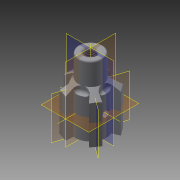
# Autodesk Inventor part: RadAxe
Saved by Autodesk Inventor 2015 (Build 190159000, 159)
## iProperties
Created: 2018-11-03
Part Number: RadAxe
Material: Generisch
Document SubType Name: Modeling
Designer: Boris
Density: 1 g/cm^3
Appearance: Vorgabe
Author: Boris
Autodesk Inventor part; units mm, degrees
sketch "Skizze1" plane through (0, 0, 0) normal (0, 0, 1) x (1, 0, 0)
  line L0 (0, -50.4) -> (0, 50.4)
  line L1 (50.4, 0) -> (-50.4, 0)
  line L2 (-7, 1.5) -> (-4.7724, 1)
  line L3 (-7, -1.5) -> (-4.7724, -1)
  line L4 (-7, -1.5) -> (-7, 1.5)
  line L5 (-0.7365, -7.1209) -> (-3.5897, -6.1939)
  line L6 (-0.7365, -7.1209) -> (-0.5237, -4.8478)
  line L7 (-3.5897, -6.1939) -> (-2.4258, -4.2298)
  line L8 (6.5448, -2.901) -> (4.7814, -5.328)
  line L9 (6.5448, -2.901) -> (4.4487, -1.9961)
  line L10 (4.7814, -5.328) -> (3.2731, -3.6141)
  line L11 (4.7814, 5.328) -> (6.5448, 2.901)
  line L12 (4.7814, 5.328) -> (3.2731, 3.6141)
  line L13 (6.5448, 2.901) -> (4.4487, 1.9961)
  line L14 (-3.5897, 6.1939) -> (-0.7365, 7.1209)
  line L15 (-3.5897, 6.1939) -> (-2.4258, 4.2298)
  line L16 (-0.7365, 7.1209) -> (-0.5237, 4.8478)
  arc A0 (-4.7724, -1) -> (-2.4258, -4.2298) centre (0, 0) ccw
  arc A1 (-0.5237, -4.8478) -> (3.2731, -3.6141) centre (0, 0) ccw
  arc A2 (4.4487, -1.9961) -> (4.4487, 1.9961) centre (0, 0) ccw
  arc A3 (3.2731, 3.6141) -> (-0.5237, 4.8478) centre (0, 0) ccw
  arc A4 (-2.4258, 4.2298) -> (-4.7724, 1) centre (0, 0) ccw
  dimension "d2" = 3
  dimension "d3" = 2
  dimension "d4" = 360
  constraints: 34 end point, 10 point on circle, 5 centre point, 2 symmetric about line, 1 coincident, 1 vertical, 36 other
  measures "d2" distance of L2.start L3.start
  measures "d3" distance of L3.end L2.end
extrude "Extrusion1" add sketch "Skizze1" along normal blind 5.407 and the other way blind 6.593
ref_plane "Arbeitsebene1" through (0.1417, -0.103, 5.407) normal (0.5877853, 0.809017, 0) x (0, 0, -1)
sketch "Skizze2" plane through (0.1417, -0.103, 5.407) normal (0.5877853, 0.809017, 0) x (0, 0, -1)
  line L0 (5.407, -13.171) -> (5.407, 13.8897) projected
  line L1 (5.407, 6.3073) -> (6.407, 6.3073)
  line L2 (6.407, 6.3073) -> (6.407, -3.6927)
  line L3 (6.407, -3.6927) -> (5.407, -3.6927)
  point P0 (5.407, 0.1752)
  dimension "d9" = 1
  dimension "d10" = 10
  constraints: 6 end point, 2 point on line, 1 horizontal, 1 parallel, 1 perpendicular
  measures "d9" distance of L2.end L3.end
  measures "d10" distance of L1.end L2.end
revolve "Umdrehung1" cut sketch "Skizze2" angle 360 about axis through (0, 0, 0) along (-0.809017, 0.5877853, 0)
ref_plane "Arbeitsebene2" through (-0.0541, -0.1666, 5.407) normal (0.9510565, -0.309017, 0) x (0, 0, -1)
mirror "Spiegeln1" about plane through (-0.0541, -0.1666, 5.407) normal (0.9510565, -0.309017, 0) of "Umdrehung1"
sketch "Skizze3" plane through (0, 0, 5.407) normal (0, 0, 1) x (1, 0, 0)
  circle A0 centre (0, 0) radius 3.75
  dimension "d12" = 7.5
  constraints: 1 centre point, 1 coincident
  measures "d12" diameter of A0
extrude "Extrusion2" add sketch "Skizze3" along normal blind 9
sketch "Skizze4" plane through (0, 0, 0) normal (0, 1, 0) x (-1, 0, 0)
  line L0 (3.75, 5.407) -> (3.75, 14.407) projected
  line L1 (7, 5.407) -> (3.75, 5.407)
  line L2 (4.7724, 5.407) -> (2.4258, 5.407) projected
  line L3 (3.75, 5.407) -> (3.75, 7.407)
  line L4 (0, -2.8814) -> (0, 17.2884) projected
  line L5 (3.75, 7.407) -> (7, 7.407)
  line L6 (7, 7.407) -> (7, 5.407)
  point P0 (0, 0)
  dimension "d15" = 2
  constraints: 8 end point, 1 collinear, 1 horizontal, 1 perpendicular, 1 point on line
  measures "d15" distance of L0.start L3.end
revolve "Umdrehung2" add sketch "Skizze4" angle 25 mid plane about axis through (0, 0, -10) along (0, 0, 1)
sketch "Skizze5" plane through (0, 0, 7.407) normal (0, 0, 1) x (1, 0, 0)
  arc A0 (-7, 0) -> (-6.8341, -1.5151) centre (0, 0) ccw
  line L0 (-7, 0) -> (-7, -1.552)
  line L1 (-6.8341, -1.5151) -> (-7, -1.552)
  point P0 (0, 0)
  point P1 (-4.7604, 1.0554)
  point P2 (-3.6611, 0.8116)
  constraints: 4 end point, 2 point on circle, 1 centre point, 1 tangent
extrude "Extrusion3" add sketch "Skizze5" against normal up to surface (2 mm away) from surface at 0
mirror "Spiegeln2" about plane through (0, 0, 0) normal (0, 1, 0) of "Extrusion3"
sketch "Skizze6" plane through (0, 0, 0) normal (0, 1, 0) x (-1, 0, 0)
  line L0 (3.6611, 5.407) -> (3.6611, 7.407) projected
  line L1 (3.75, 7.407) -> (3.75, 14.407) projected
  line L2 (0, -10.793) -> (0, 18.607) projected
  line L3 (3.75, 7.407) -> (7.6989, 4.9769)
  line L4 (3.75, 7.407) -> (7.6989, 7.407)
  line L5 (7.6989, 7.407) -> (7.6989, 4.9769)
  point P0 (0, 0)
  point P1 (7, 7.407)
  point P2 (7, 5.407)
  constraints: 6 end point, 1 horizontal, 1 perpendicular, 1 point on line
pattern_circular "Runde Anordnung1" count 5 over 360 about axis through (0, 0, 5.407) along (0, 0, 1) of "Umdrehung2", "Extrusion3", "Spiegeln2"
revolve "Umdrehung4" cut sketch "Skizze6" angle 360 about axis through (0, 0, -10) along (0, 0, 1)
sketch "Skizze7" plane through (0, 0, -6.593) normal (0, 0, -1) x (-1, 0, 0)
  line L0 (7, 1.5) -> (4.7724, 1) projected
  arc A0 (4.7724, 1) -> (2.4258, 4.2298) centre (0, 0) ccw projected
  line L1 (2.4258, 4.2298) -> (3.5897, 6.1939) projected
  line L2 (3.5897, 6.1939) -> (0.7365, 7.1209) projected
  line L3 (0.7365, 7.1209) -> (0.5237, 4.8478) projected
  arc A1 (0.5237, 4.8478) -> (-3.2731, 3.6141) centre (0, 0) ccw projected
  line L4 (-3.2731, 3.6141) -> (-4.7814, 5.328) projected
  line L5 (-4.7814, 5.328) -> (-6.5448, 2.901) projected
  line L6 (-6.5448, 2.901) -> (-4.4487, 1.9961) projected
  arc A2 (-4.4487, 1.9961) -> (-4.4487, -1.9961) centre (0, 0) ccw projected
  line L7 (-4.4487, -1.9961) -> (-6.5448, -2.901) projected
  line L8 (-6.5448, -2.901) -> (-4.7814, -5.328) projected
  line L9 (-4.7814, -5.328) -> (-3.2731, -3.6141) projected
  arc A3 (-3.2731, -3.6141) -> (0.5237, -4.8478) centre (0, 0) ccw projected
  line L10 (0.5237, -4.8478) -> (0.7365, -7.1209) projected
  line L11 (0.7365, -7.1209) -> (3.5897, -6.1939) projected
  line L12 (3.5897, -6.1939) -> (2.4258, -4.2298) projected
  arc A4 (2.4258, -4.2298) -> (4.7724, -1) centre (0, 0) ccw projected
  line L13 (4.7724, -1) -> (7, -1.5) projected
  line L14 (7, -1.5) -> (7, 1.5) projected
  arc A5 (4.8161, -4.6696) -> (5.9293, -3.1375) centre (0, 0) ccw
  line L15 (4.8161, -4.6696) -> (6.3329, -7.229)
  line L16 (6.3329, -7.229) -> (-0.8743, -9.5708)
  line L17 (-0.8743, -9.5708) -> (-1.1517, -6.6086)
  arc A6 (-2.9527, -6.0234) -> (-1.1517, -6.6086) centre (0, 0) ccw
  line L18 (-2.9527, -6.0234) -> (-4.9183, -8.2568)
  line L19 (-4.9183, -8.2568) -> (-9.3725, -2.126)
  line L20 (-9.3725, -2.126) -> (-6.641, -0.9469)
  arc A7 (-6.641, 0.9469) -> (-6.641, -0.9469) centre (0, 0) ccw
  line L21 (-6.641, 0.9469) -> (-9.3725, 2.126)
  line L22 (-9.3725, 2.126) -> (-4.9183, 8.2568)
  line L23 (-4.9183, 8.2568) -> (-2.9527, 6.0234)
  arc A8 (-1.1517, 6.6086) -> (-2.9527, 6.0234) centre (0, 0) ccw
  line L24 (-1.1517, 6.6086) -> (-0.8743, 9.5708)
  line L25 (-0.8743, 9.5708) -> (6.3329, 7.229)
  line L26 (6.3329, 7.229) -> (4.8161, 4.6696)
  arc A9 (5.9293, 3.1375) -> (4.8161, 4.6696) centre (0, 0) ccw
  line L27 (5.9293, 3.1375) -> (8.8322, 3.789)
  line L28 (8.8322, 3.789) -> (8.8322, -3.789)
  line L29 (8.8322, -3.789) -> (5.9293, -3.1375)
  constraints: 30 end point, 10 point on circle, 5 centre point, 19 other
extrude "Extrusion4" cut sketch "Skizze7" against normal blind 20
fillet "Rundung1" radius 2 10 edges at (2.4848, -2.8086, 6.407) (-0.3594, -3.7327, 6.407) (-1.9033, -3.2311, 6.407) (-3.6611, -0.8116, 6.407) (-3.6611, 0.8116, 6.407) (-1.9033, 3.2311, 6.407) (-0.3594, 3.7327, 6.407) (3.439, -1.4953, 6.407) (2.4848, 2.8086, 6.407) (3.439, 1.4953, 6.407)
fillet "Rundung2" radius 1 16 edges at (3.7478, 0.1289, 5.407) (3.7478, -0.1289, 5.407) (3.9011, 1.1899, 5.407) (3.9011, -1.1899, 5.407) (1.1588, -3.5665, 5.407) (0.0739, -4.0779, 5.407) (2.3371, -3.3425, 5.407) (-3.0338, -2.2042, 5.407) (-3.8555, -1.3304, 5.407) (-2.4567, -3.2556, 5.407) (-3.0338, 2.2042, 5.407) (-3.8555, 1.3304, 5.407) (-2.4567, 3.2556, 5.407) (1.1588, 3.5665, 5.407) (2.3371, 3.3425, 5.407) (0.0739, 4.0779, 5.407)
sketch "Skizze8" plane through (0, 0, 14.407) normal (0, 0, 1) x (1, 0, 0)
  circle A0 centre (0, 0) radius 1.5
  dimension "d28" = 3
  constraints: 1 centre point, 1 coincident
  measures "d28" diameter of A0
extrude "Extrusion5" cut sketch "Skizze8" against normal blind 13
thread "Gewinde1" size "M3x0.5" class "6H" standard "ANSI Metric M Profile" full length
fillet "Rundung3" radius 0.5 1 edges at (-3.75, 0, 14.407)
fillet "Rundung4" radius 1 1 edges at (-1.5, 0, 14.407)
